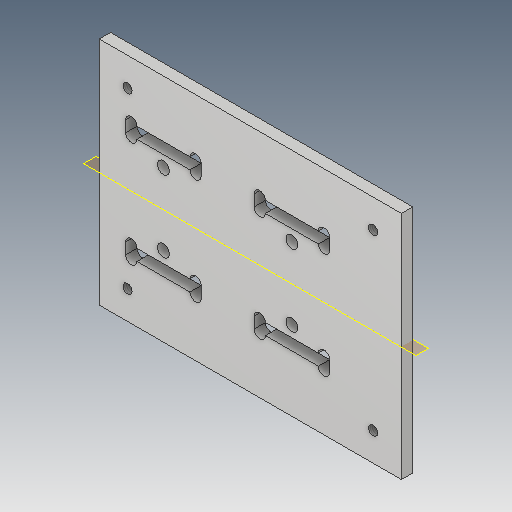
# Autodesk Inventor part: plate2
Saved by Autodesk Inventor 2019.4 (Build 234330000, 330)
## iProperties
Created: 2019-06-29
Part Number: plate2
Material: アルミニウム 2014-T4
Document SubType Name: Modeling
Designer: AzLIer
Density: 2.8 g/cm^3
Appearance: サテン
Author: AzLIer
Autodesk Inventor part; units mm, degrees
ref_plane "YZ Plane" through (0, 0, 0) normal (1, 0, 0) x (0, 1, 0)
ref_plane "XZ Plane" through (0, 0, 0) normal (0, 1, 0) x (-1, 0, 0)
ref_plane "XY Plane" through (0, 0, 0) normal (0, 0, 1) x (1, 0, 0)
sketch "スケッチ1" plane through (0, 0, 0) normal (0, 0, 1) x (1, 0, 0)
  line L0 (0, -31) -> (0, -46) projected
  line L1 (0, -31) -> (-140, -31) projected
  line L2 (-140, -46) -> (-140, -31) projected
  line L3 (0, -46) -> (-140, -46) projected
  line L4 (-30, 15) -> (-110, 15)
  line L5 (-110, 15) -> (-110, -46)
  line L6 (-110, -46) -> (-30, -46)
  line L7 (-30, -46) -> (-30, 15)
  line L8 (0, 15) -> (0, 0) projected
  line L9 (0, 15) -> (-140, 15) projected
  line L10 (-140, 0) -> (-140, 15) projected
  line L11 (0, 0) -> (-140, 0) projected
  circle A0 centre (-37.5, 7.5) radius 1.6 projected
  circle A1 centre (-102.5, 7.5) radius 1.6 projected
  circle A2 centre (-37.5, -38.5) radius 1.6 projected
  circle A3 centre (-102.5, -38.5) radius 1.6 projected
  dimension "d1" = 80
  dimension "d15" = 30
  constraints: 8 end point, 2 parallel, 2 point on line, 1 horizontal, 1 perpendicular
  measures "d1" distance between parallel lines of L5 L7
  measures "d15" distance between parallel lines of L8 L7
extrude "押し出し1" add sketch "スケッチ1" along normal blind 3 contours L7 L3 L5 L1 | L1 L5 L11 L7 | L11 L5 L4 L7 | A0 | A1 | A2 | A3
sketch "スケッチ2" plane through (0, 0, 3) normal (0, 0, 1) x (1, 0, 0)
  line L0 (-110, -46) -> (-30, -46) projected
  line L1 (-30, 15) -> (-110, 15) projected
  line L2 (-30, -46) -> (-30, 15) projected
  line L3 (-110, 15) -> (-110, -46) projected
  point P0 (0, 0)
  point P1 (-37.5, 7.5)
  point P2 (-37.5, -38.5)
  point P3 (-102.5, -38.5)
  point P4 (-102.5, 7.5)
  dimension "d4" = 7.5
  dimension "d5" = 7.5
  dimension "d6" = 7.5
  dimension "d7" = 7.5
  constraints: 2 horizontal alignment, 2 vertical alignment
  measures "d4" distance from line of L0 point (-37.5, -38.5)
  measures "d5" distance from line of L1 point (-37.5, 7.5)
  measures "d6" distance from line of L2 point (-37.5, -38.5)
  measures "d7" distance from line of L3 point (-102.5, -38.5)
hole "穴1" at (-37.5, 7.5, 3) at (-37.5, -38.5, 3) at (-102.5, -38.5, 3) at (-102.5, 7.5, 3) direction (0, 0, -1) diameter 2.459 end through all thread size "M3x0.5" class "6H" standard "ISO Metric profile"
sketch "スケッチ3" plane through (0, 0, 3) normal (0, 0, 1) x (1, 0, 0)
  line L0 (-52, -28) -> (-66, -28)
  line L1 (-69, -28) -> (-69, -31)
  line L2 (-52, -31) -> (-66, -31)
  line L3 (-49, -28) -> (-49, -31)
  line L4 (-30, -46) -> (-30, 15) projected
  line L5 (-110, -46) -> (-30, -46) projected
  arc A0 (-69, -31) -> (-66, -31) centre (-67.5, -31) ccw
  arc A1 (-52, -31) -> (-49, -31) centre (-50.5, -31) ccw
  arc A2 (-66, -28) -> (-69, -28) centre (-67.5, -28) ccw
  arc A3 (-49, -28) -> (-52, -28) centre (-50.5, -28) ccw
  circle A4 centre (-59, -25) radius 1.6
  point P0 (0, 0)
  point P1 (-59, -28)
  dimension "d16" = 19
  dimension "d17" = 15
  dimension "d18" = 3
  dimension "d19" = 20
  dimension "d21" = 3
  dimension "d32" = 3
  dimension "d33" = 3.2
  constraints: 8 end point, 8 point on circle, 8 point on line, 5 centre point, 3 equal radius, 1 midpoint, 1 parallel, 1 tangent, 1 vertical alignment
  measures "d16" distance between parallel lines of L4 L3
  measures "d17" distance between parallel lines of L5 L2
  measures "d18" distance of L3.start L3.end
  measures "d19" distance of L3.end L1.end
  measures "d21" diameter of A1
  measures "d32" distance from line of L0 A4.centre
  measures "d33" diameter of A4
extrude "押し出し2" cut sketch "スケッチ3" against normal blind 3
ref_plane "作業平面1" through (-110, -15.5, 0) normal (0, 1, 0) x (1, 0, 0)
mirror "ミラー1" about plane through (-110, -15.5, 0) normal (0, 1, 0) of "押し出し2"
pattern_linear "矩形状パターン1" count 2 spacing 34 along (-1, 0, 0) of "押し出し2", "ミラー1"
equation "\"d5\" = d4"
